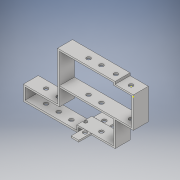
# Autodesk Inventor part: SENGH IS KENGH
Saved by Autodesk Inventor 2017 (Build 210142000, 142)
## iProperties
Created: 2017-11-30
Part Number: SENGH IS KENGH
Material: Generic
Document SubType Name: Modeling
Designer: Sam
Density: 1 g/cm^3
Appearance: Default
Author: Sam
Autodesk Inventor part; units mm, degrees
ref_plane "YZ Plane" through (0, 0, 0) normal (1, 0, 0) x (0, 1, 0)
ref_plane "XZ Plane" through (0, 0, 0) normal (0, 1, 0) x (-1, 0, 0)
ref_plane "XY Plane" through (0, 0, 0) normal (0, 0, 1) x (1, 0, 0)
sketch "Sketch1" plane through (0, 0, 0) normal (0, 0, 1) x (1, 0, 0)
  line L0 (0, 2) -> (0, 0) projected
  line L1 (0, 2) -> (-89, 2) projected
  line L2 (-89, 0) -> (-89, 2) projected
  line L3 (0, 0) -> (-89, 0) projected
  circle A0 centre (-28, -35.5) radius 1.5 projected
  circle A1 centre (-36, -35.5) radius 1.5 projected
  line L4 (-66, -36) -> (-40, -36) projected
  line L5 (-40, -36) -> (-40, -41) projected
  line L6 (-20.7846, -41) -> (-40, -41) projected
  line L7 (-20.7846, 0) -> (-20.7846, -41) projected
  line L8 (-20.7846, 0) -> (-22, 0) projected
  line L9 (-22, 0) -> (-22, -30) projected
  line L10 (-66, -31.5748) -> (-66, -36) projected
  line L11 (0, -41) -> (-20.7846, -41) projected
  line L12 (0, 0) -> (0, -41) projected
  line L13 (0, 0) -> (-20.7846, 0) projected
  line L14 (-20.7846, 0) -> (-20.7846, -41) projected
  line L15 (0, 46) -> (0, 0) projected
  circle A2 centre (-28, 45.5) radius 1.5 projected
  circle A3 centre (-36, 45.5) radius 1.5 projected
  circle A4 centre (-98, 52) radius 1.5 projected
  line L16 (-49.0437, 51) -> (-20.7846, 51) projected
  line L17 (-104, 55.8081) -> (-49.0437, 51) projected
  line L18 (-104, 55.8081) -> (-104, 48) projected
  line L19 (-104, 48) -> (-81, 48) projected
  line L20 (-81, 48) -> (-81, 42.8871) projected
  line L21 (-81, 42.8871) -> (-48, 40) projected
  line L22 (-48, 40) -> (-22, 40) projected
  line L23 (-22, 40) -> (-22, 46) projected
  line L24 (-22, 46) -> (-20.7846, 46) projected
  line L25 (-20.7846, 51) -> (-20.7846, 46) projected
  line L26 (-22, 46) -> (0, 46) projected
  line L27 (-22, 40) -> (-22, 46) projected
  line L28 (0, 40) -> (-22, 40) projected
  line L29 (0, 46) -> (0, 40) projected
  line L30 (-22, 0) -> (-22, -30)
  line L31 (-91.246, 40) -> (-22, 40)
  line L32 (-22, 40) -> (-22, 36.9892)
  line L33 (-22, 36.9892) -> (0, 36.9892)
  line L34 (0, 36.9892) -> (0, 2)
  line L35 (-23.9878, 0) -> (-24, 0)
  line L36 (-24, 0) -> (-23.8812, -27.9971)
  line L37 (-91, -18) -> (-114, -18) projected
  line L38 (-132.3701, 81.1945) -> (-132.3701, -67.1672)
  line L39 (-91, -18) -> (-132.3701, -18)
  line L40 (-132.3701, -18) -> (-132.3701, -29.4267)
  line L41 (-91, -18) -> (-91.246, 40)
  line L42 (-23.8812, -27.9971) -> (-68.0077, -28.1843)
  line L43 (-130.363, -20.001) -> (-88.993, -20.001)
  line L44 (-88.993, 37.9938) -> (-23.9878, 37.9938)
  line L45 (-23.9878, 37.9938) -> (-23.9878, 35.1472)
  line L46 (-23.9878, 35.1472) -> (-2.1372, 35.1472)
  line L47 (-2.1372, 35.1472) -> (-2.1372, 2)
  line L48 (-130.363, -20.001) -> (-130.363, -33.7874)
  line L49 (-130.363, -36) -> (-66, -36)
  line L50 (-132.3701, -18) -> (-132.3701, -36)
  line L51 (-132.3701, -36) -> (-130.363, -36)
  line L52 (-130.363, -33.7874) -> (-68, -33.7874)
  line L53 (-66, -33.7874) -> (-66, -36)
  line L54 (-66, -33.7874) -> (-66, -31.5748)
  line L55 (-68, -33.7874) -> (-68, -31.5748)
  line L56 (-68, -31.5748) -> (-68, -30)
  line L57 (-68, -30) -> (-68.0077, -28.1843)
  line L58 (-66, -30.1103) -> (-66, -31.5748)
  line L59 (-22, -30) -> (-66, -30)
  line L60 (-66, -30) -> (-66, -30.1103)
  line L61 (-2.1372, 2) -> (-89, 2)
  line L62 (0, 2) -> (0, 0)
  line L63 (0, 0) -> (-22, 0)
  line L64 (-24, 0) -> (-89, 0)
  line L65 (-88.993, -20.001) -> (-88.993, 0)
  line L66 (-88.993, 2) -> (-88.993, 37.9938)
  dimension "d0" = 2
  dimension "d1" = 27.9974
  dimension "d6" = 41.37
  dimension "d8" = 57.9948
  dimension "d10" = 65.0052
  dimension "d14" = 2
  constraints: 72 end point, 13 perpendicular, 11 point on line, 6 vertical, 4 collinear, 2 parallel, 1 horizontal, 1 midpoint, 2 other
  measures "d0" distance of L8.end L35.end
  measures "d1" distance of L35.end L36.end
  measures "d6" distance of L43.start L43.end
  measures "d8" distance of L43.end L44.start
  measures "d10" distance of L44.start L44.end
  measures "d14" distance of L52.end L53.start
extrude "Extrusion2" add sketch "Sketch1" against normal blind 18 contours L1 L47 L46 L45 L44 L66 L2 L3 L65 L43 L48 L52 L55 L56 L57 L42 L36 L9 L59 L60 L58 L10 L49 L51 L38 L39 L37 L41 L31 L22 L32 L33 L15
sketch "Sketch5" plane through (-23.9878, 35.1472, 0) normal (0, -1, 0) x (1, 0, 0)
  point P0 (23.9878, 0)
sketch "Sketch6" plane through (0, 0, -18) normal (0, 0, -1) x (-1, 0, 0)
  line L0 (22, -30) -> (66, -30) projected
  line L1 (68.0077, -28.1843) -> (23.8812, -27.9971) projected
  line L2 (66, -30) -> (46.9738, -30)
  line L3 (46.9738, -30) -> (46.9738, -28.0951)
  line L4 (46.9738, -28.0951) -> (66, -28.0951)
  line L5 (66, -28.0951) -> (66, -30)
  point P0 (0, 0)
  constraints: 8 end point, 2 parallel, 1 horizontal, 1 perpendicular, 1 point on line
extrude "Extrusion6" add sketch "Sketch6" along normal blind 25
sketch "Sketch7" plane through (-132.3701, -36, 0) normal (0, -1, 0) x (1, 0, 0)
  arc A0 (20.1763, -7.9629) -> (20.3806, -9.5438) centre (18.3701, -9) ccw
  spline S0 degree 3 number of poles 884
  arc A1 (63.5787, -11.8624) -> (67.8965, -12.5067) centre (66.2955, -8.4452) ccw
  arc A2 (67.8965, -12.5067) -> (70.6134, -9.0895) centre (66.2955, -8.4452) ccw
  arc A3 (70.6134, -9.0895) -> (69.0124, -5.028) centre (66.2955, -8.4452) ccw
  arc A4 (69.0124, -5.028) -> (64.6946, -4.3837) centre (66.2955, -8.4452) ccw
  arc A5 (64.6946, -4.3837) -> (61.9777, -7.8009) centre (66.2955, -8.4452) ccw
  arc A6 (61.9777, -7.8009) -> (63.5787, -11.8624) centre (66.2955, -8.4452) ccw
  arc A7 (67.9695, -7.2059) -> (66.6029, -6.3852) centre (66.2955, -8.4452) ccw
  arc A8 (66.6029, -6.3852) -> (67.9695, -7.2059) centre (66.2955, -8.4452) ccw
  arc A9 (73.8571, -24.1243) -> (78.1749, -24.7686) centre (76.574, -20.7071) ccw
  arc A10 (78.1749, -24.7686) -> (80.8918, -21.3514) centre (76.574, -20.7071) ccw
  arc A11 (80.8918, -21.3514) -> (79.2908, -17.2899) centre (76.574, -20.7071) ccw
  arc A12 (79.2908, -17.2899) -> (74.973, -16.6456) centre (76.574, -20.7071) ccw
  arc A13 (74.973, -16.6456) -> (72.2561, -20.0628) centre (76.574, -20.7071) ccw
  arc A14 (72.2561, -20.0628) -> (73.8571, -24.1243) centre (76.574, -20.7071) ccw
  arc A15 (78.2479, -19.4678) -> (76.8813, -18.6471) centre (76.574, -20.7071) ccw
  arc A16 (76.8813, -18.6471) -> (78.2479, -19.4678) centre (76.574, -20.7071) ccw
  spline S1 degree 3 number of poles 1000
  arc A17 (69.1532, -39.4172) -> (73.471, -40.0615) centre (71.8701, -36) ccw
  arc A18 (73.471, -40.0615) -> (76.1879, -36.6443) centre (71.8701, -36) ccw
  arc A19 (76.1879, -36.6443) -> (74.5869, -32.5828) centre (71.8701, -36) ccw
  arc A20 (74.5869, -32.5828) -> (70.2691, -31.9385) centre (71.8701, -36) ccw
  arc A21 (70.2691, -31.9385) -> (67.5522, -35.3557) centre (71.8701, -36) ccw
  arc A22 (67.5522, -35.3557) -> (69.1532, -39.4172) centre (71.8701, -36) ccw
  arc A23 (73.544, -34.7607) -> (72.1774, -33.94) centre (71.8701, -36) ccw
  arc A24 (72.1774, -33.94) -> (73.544, -34.7607) centre (71.8701, -36) ccw
  point P0 (132.3701, 0)
sketch "Sketch8" plane through (0, 0, 0) normal (0, 0, 1) x (1, 0, 0)
  line L0 (0, 2) -> (0, 36.9892) projected
  line L1 (0, 2) -> (-88.993, 2)
  line L2 (-88.993, 2) -> (-88.993, 0)
  line L3 (-88.993, 0) -> (0, 0)
  line L4 (0, 0) -> (0, 2)
  point P0 (0, 0)
  constraints: 8 end point, 2 parallel, 1 horizontal, 1 perpendicular
extrude "Extrusion7" add sketch "Sketch8" against normal blind 18
sketch "Sketch9" plane through (-23.9878, 35.1472, 0) normal (0, -1, 0) x (1, 0, 0)
  circle A0 centre (12.9653, -8.5) radius 1 projected
  point P0 (23.9878, 0)
sketch "Sketch10" plane through (-22, 36.9892, 0) normal (0, 1, 0) x (1, 0, 0)
  circle A0 centre (10.6789, 8.5163) radius 2.5
  point P0 (22, 0)
  dimension "d27" = 5
  constraints: 1 centre point
  measures "d27" diameter of A0
sketch "Sketch11" plane through (-23.9878, 35.1472, 0) normal (0, -1, 0) x (1, 0, 0)
  point P0 (23.9878, 0)
extrude "Extrusion8" cut sketch "Sketch10" against normal through all
sketch "Sketch12" plane through (-132.3701, -36, 0) normal (0, -1, 0) x (1, 0, 0)
  circle A0 centre (18.3329, -9.0632) radius 2.5
  circle A1 centre (66.3878, -8.536) radius 2.5
  point P0 (132.3701, 0)
  dimension "d30" = 5
  dimension "d31" = 5
  constraints: 2 centre point
  measures "d30" diameter of A0
  measures "d31" diameter of A1
extrude "Extrusion9" cut sketch "Sketch12" against normal through all contours A0
extrude "Extrusion10" cut sketch "Sketch7" against normal blind 25 contours A8 A7
sketch "Sketch14" plane through (-132.3701, -36, 0) normal (0, -1, 0) x (1, 0, 0)
  arc A0 (47.613, -10.8143) -> (51.9308, -11.4586) centre (50.3299, -7.3971) ccw projected
  arc A1 (51.9308, -11.4586) -> (54.6477, -8.0414) centre (50.3299, -7.3971) ccw projected
  arc A2 (54.6477, -8.0414) -> (53.0468, -3.9799) centre (50.3299, -7.3971) ccw projected
  arc A3 (53.0468, -3.9799) -> (48.7289, -3.3356) centre (50.3299, -7.3971) ccw projected
  arc A4 (48.7289, -3.3356) -> (46.0121, -6.7528) centre (50.3299, -7.3971) ccw projected
  arc A5 (46.0121, -6.7528) -> (47.613, -10.8143) centre (50.3299, -7.3971) ccw projected
  arc A6 (52.0039, -6.1578) -> (50.6373, -5.3371) centre (50.3299, -7.3971) ccw projected
  arc A7 (50.6373, -5.3371) -> (52.0039, -6.1578) centre (50.3299, -7.3971) ccw projected
  circle A8 centre (50.3299, -7.3971) radius 2.5
  point P0 (132.3701, 0)
  dimension "d39" = 5
  constraints: 1 centre point, 1 coincident
  measures "d39" diameter of A8
extrude "Extrusion12" cut sketch "Sketch14" against normal blind 5 contours A7 A6 | A8
sketch "Sketch15" plane through (-66, -30, 0) normal (0, -1, 0) x (1, 0, 0)
  circle A0 centre (19.9882, -7.5812) radius 1.4875 projected
  arc A1 (7.487, -24.1243) -> (11.8049, -24.7686) centre (10.2039, -20.7071) ccw projected
  arc A2 (11.8049, -24.7686) -> (14.5217, -21.3514) centre (10.2039, -20.7071) ccw projected
  arc A3 (14.5217, -21.3514) -> (12.9208, -17.2899) centre (10.2039, -20.7071) ccw projected
  arc A4 (12.9208, -17.2899) -> (8.6029, -16.6456) centre (10.2039, -20.7071) ccw projected
  arc A5 (8.6029, -16.6456) -> (5.8861, -20.0628) centre (10.2039, -20.7071) ccw projected
  arc A6 (5.8861, -20.0628) -> (7.487, -24.1243) centre (10.2039, -20.7071) ccw projected
  arc A7 (11.8779, -19.4678) -> (10.5113, -18.6471) centre (10.2039, -20.7071) ccw projected
  arc A8 (10.5113, -18.6471) -> (11.8779, -19.4678) centre (10.2039, -20.7071) ccw projected
  arc A9 (2.7831, -39.4172) -> (7.101, -40.0615) centre (5.5, -36) ccw projected
  arc A10 (7.101, -40.0615) -> (9.8178, -36.6443) centre (5.5, -36) ccw projected
  arc A11 (9.8178, -36.6443) -> (8.2169, -32.5828) centre (5.5, -36) ccw projected
  arc A12 (8.2169, -32.5828) -> (3.899, -31.9385) centre (5.5, -36) ccw projected
  arc A13 (3.899, -31.9385) -> (1.1822, -35.3557) centre (5.5, -36) ccw projected
  arc A14 (1.1822, -35.3557) -> (2.7831, -39.4172) centre (5.5, -36) ccw projected
  arc A15 (7.174, -34.7607) -> (5.8074, -33.94) centre (5.5, -36) ccw projected
  arc A16 (5.8074, -33.94) -> (7.174, -34.7607) centre (5.5, -36) ccw projected
  circle A17 centre (19.9882, -7.5812) radius 2.5
  circle A18 centre (10.2039, -20.7071) radius 2.5
  circle A19 centre (5.5, -36) radius 2.5
  point P0 (66, 0)
  dimension "d42" = 5
  dimension "d43" = 5
  dimension "d44" = 5
  constraints: 3 centre point, 3 coincident
  measures "d42" diameter of A17
  measures "d43" diameter of A18
  measures "d44" diameter of A19
extrude "Extrusion13" cut sketch "Sketch15" against normal blind 50 contours A0 | A8 A7 | A16 A15 | A17 | A18 | A19
sketch "Sketch17" plane through (-91.246, 40, 0) normal (0, 1, 0) x (1, 0, 0)
  circle A0 centre (62.2283, 8.0888) radius 2.5
  arc A1 (72.7505, 5.8875) -> (75.0997, 6.2647) centre (72.5002, 14.9506) ccw
  arc A2 (72.584, 5.204) -> (72.7505, 5.8875) centre (62.2283, 8.0888) ccw
  arc A3 (74.4965, 3.7887) -> (72.584, 5.204) centre (68.1934, -2.7285) ccw
  arc A4 (74.189, 2.9955) -> (74.4965, 3.7887) centre (62.2283, 8.0888) ccw
  arc A5 (71.8222, 3.2392) -> (74.189, 2.9955) centre (73.9261, 12.0582) ccw
  arc A6 (71.4845, 2.6221) -> (71.8222, 3.2392) centre (62.2283, 8.0888) ccw
  arc A7 (72.9655, 0.76) -> (71.4845, 2.6221) centre (65.1905, -3.9038) ccw
  arc A8 (72.4632, 0.0734) -> (72.9655, 0.76) centre (62.2283, 8.0888) ccw
  arc A9 (70.2402, 0.9213) -> (72.4632, 0.0734) centre (74.5549, 8.8954) ccw
  arc A10 (69.7542, 0.4127) -> (70.2402, 0.9213) centre (62.2283, 8.0888) ccw
  arc A11 (70.7028, -1.7693) -> (69.7542, 0.4127) centre (61.9856, -4.2618) ccw
  arc A12 (70.0399, -2.3025) -> (70.7028, -1.7693) centre (62.2283, 8.0888) ccw
  arc A13 (68.1121, -0.9081) -> (70.0399, -2.3025) centre (74.3436, 5.6775) ccw
  arc A14 (67.5111, -1.2736) -> (68.1121, -0.9081) centre (62.2283, 8.0888) ccw
  arc A15 (67.8626, -3.6268) -> (67.5111, -1.2736) centre (58.7973, -3.7782) ccw
  arc A16 (67.0843, -3.9702) -> (67.8626, -3.6268) centre (62.2283, 8.0888) ccw
  arc A17 (65.583, -2.1244) -> (67.0843, -3.9702) centre (73.3067, 2.624) ccw
  arc A18 (64.9079, -2.3219) -> (65.583, -2.1244) centre (62.2283, 8.0888) ccw
  arc A19 (64.6384, -4.6859) -> (64.9079, -2.3219) centre (55.8428, -2.4858) ccw
  arc A20 (63.7977, -4.8161) -> (64.6384, -4.6859) centre (62.2283, 8.0888) ccw
  arc A21 (62.8254, -2.6446) -> (63.7977, -4.8161) centre (71.5149, -0.0571) ccw
  arc A22 (62.1221, -2.6607) -> (62.8254, -2.6446) centre (62.2283, 8.0888) ccw
  arc A23 (61.25, -4.8744) -> (62.1221, -2.6607) centre (53.3235, -0.4728) ccw
  arc A24 (60.4042, -4.7826) -> (61.25, -4.8744) centre (62.2283, 8.0888) ccw
  arc A25 (60.027, -2.4334) -> (60.4042, -4.7826) centre (69.0901, -2.1831) ccw
  arc A26 (59.3435, -2.2669) -> (60.027, -2.4334) centre (62.2283, 8.0888) ccw
  arc A27 (57.9282, -4.1794) -> (59.3435, -2.2669) centre (51.411, 2.1236) ccw
  arc A28 (57.135, -3.8719) -> (57.9282, -4.1794) centre (62.2283, 8.0888) ccw
  arc A29 (57.3787, -1.5052) -> (57.135, -3.8719) centre (66.1977, -3.6091) ccw
  arc A30 (56.7616, -1.1675) -> (57.3787, -1.5052) centre (62.2283, 8.0888) ccw
  arc A31 (54.8995, -2.6485) -> (56.7616, -1.1675) centre (50.2357, 5.1266) ccw
  arc A32 (54.2129, -2.1461) -> (54.8995, -2.6485) centre (62.2283, 8.0888) ccw
  arc A33 (55.0608, 0.0769) -> (54.2129, -2.1461) centre (63.0349, -4.2378) ccw
  arc A34 (54.5522, 0.5628) -> (55.0608, 0.0769) centre (62.2283, 8.0888) ccw
  arc A35 (52.3702, -0.3858) -> (54.5522, 0.5628) centre (49.8777, 8.3314) ccw
  arc A36 (51.837, 0.2771) -> (52.3702, -0.3858) centre (62.2283, 8.0888) ccw
  arc A37 (53.2314, 2.205) -> (51.837, 0.2771) centre (59.817, -4.0266) ccw
  arc A38 (52.8659, 2.806) -> (53.2314, 2.205) centre (62.2283, 8.0888) ccw
  arc A39 (50.5127, 2.4545) -> (52.8659, 2.806) centre (50.3613, 11.5197) ccw
  arc A40 (50.1693, 3.2328) -> (50.5127, 2.4545) centre (62.2283, 8.0888) ccw
  arc A41 (52.0151, 4.734) -> (50.1693, 3.2328) centre (56.7635, -2.9897) ccw
  arc A42 (51.8176, 5.4092) -> (52.0151, 4.734) centre (62.2283, 8.0888) ccw
  arc A43 (49.4536, 5.6787) -> (51.8176, 5.4092) centre (51.6537, 14.4742) ccw
  arc A44 (49.3234, 6.5193) -> (49.4536, 5.6787) centre (62.2283, 8.0888) ccw
  arc A45 (51.4949, 7.4917) -> (49.3234, 6.5193) centre (54.0824, -1.1978) ccw
  arc A46 (51.4788, 8.195) -> (51.4949, 7.4917) centre (62.2283, 8.0888) ccw
  arc A47 (49.2651, 9.0671) -> (51.4788, 8.195) centre (53.6667, 16.9936) ccw
  arc A48 (49.3569, 9.9128) -> (49.2651, 9.0671) centre (62.2283, 8.0888) ccw
  arc A49 (51.7061, 10.29) -> (49.3569, 9.9128) centre (51.9564, 1.227) ccw
  arc A50 (51.8726, 10.9735) -> (51.7061, 10.29) centre (62.2283, 8.0888) ccw
  arc A51 (49.9601, 12.3889) -> (51.8726, 10.9735) centre (56.2631, 18.906) ccw
  arc A52 (50.2676, 13.182) -> (49.9601, 12.3889) centre (62.2283, 8.0888) ccw
  arc A53 (52.6343, 12.9384) -> (50.2676, 13.182) centre (50.5304, 4.1193) ccw
  arc A54 (52.972, 13.5555) -> (52.6343, 12.9384) centre (62.2283, 8.0888) ccw
  arc A55 (51.491, 15.4176) -> (52.972, 13.5555) centre (59.2661, 20.0813) ccw
  arc A56 (51.9934, 16.1042) -> (51.491, 15.4176) centre (62.2283, 8.0888) ccw
  arc A57 (54.2164, 15.2562) -> (51.9934, 16.1042) centre (49.9017, 7.2822) ccw
  arc A58 (54.7023, 15.7649) -> (54.2164, 15.2562) centre (62.2283, 8.0888) ccw
  arc A59 (53.7537, 17.9469) -> (54.7023, 15.7649) centre (62.4709, 20.4394) ccw
  arc A60 (54.4166, 18.48) -> (53.7537, 17.9469) centre (62.2283, 8.0888) ccw
  arc A61 (56.3445, 17.0856) -> (54.4166, 18.48) centre (50.1129, 10.5) ccw
  arc A62 (56.9455, 17.4512) -> (56.3445, 17.0856) centre (62.2283, 8.0888) ccw
  arc A63 (56.594, 19.8043) -> (56.9455, 17.4512) centre (65.6592, 19.9557) ccw
  arc A64 (57.3723, 20.1478) -> (56.594, 19.8043) centre (62.2283, 8.0888) ccw
  arc A65 (58.8735, 18.3019) -> (57.3723, 20.1478) centre (51.1498, 13.5536) ccw
  arc A66 (59.5487, 18.4995) -> (58.8735, 18.3019) centre (62.2283, 8.0888) ccw
  arc A67 (59.8182, 20.8634) -> (59.5487, 18.4995) centre (68.6137, 18.6634) ccw
  arc A68 (60.6588, 20.9937) -> (59.8182, 20.8634) centre (62.2283, 8.0888) ccw
  arc A69 (61.6312, 18.8222) -> (60.6588, 20.9937) centre (52.9417, 16.2347) ccw
  arc A70 (62.3345, 18.8383) -> (61.6312, 18.8222) centre (62.2283, 8.0888) ccw
  arc A71 (63.2066, 21.0519) -> (62.3345, 18.8383) centre (71.1331, 16.6504) ccw
  arc A72 (64.0523, 20.9602) -> (63.2066, 21.0519) centre (62.2283, 8.0888) ccw
  arc A73 (64.4295, 18.611) -> (64.0523, 20.9602) centre (55.3665, 18.3607) ccw
  arc A74 (65.113, 18.4445) -> (64.4295, 18.611) centre (62.2283, 8.0888) ccw
  arc A75 (66.5284, 20.357) -> (65.113, 18.4445) centre (73.0455, 14.0539) ccw
  arc A76 (67.3215, 20.0495) -> (66.5284, 20.357) centre (62.2283, 8.0888) ccw
  arc A77 (67.0779, 17.6827) -> (67.3215, 20.0495) centre (58.2588, 19.7866) ccw
  arc A78 (67.695, 17.345) -> (67.0779, 17.6827) centre (62.2283, 8.0888) ccw
  arc A79 (69.5571, 18.826) -> (67.695, 17.345) centre (74.2208, 11.051) ccw
  arc A80 (70.2437, 18.3237) -> (69.5571, 18.826) centre (62.2283, 8.0888) ccw
  arc A81 (69.3957, 16.1007) -> (70.2437, 18.3237) centre (61.4217, 20.4154) ccw
  arc A82 (69.9044, 15.6147) -> (69.3957, 16.1007) centre (62.2283, 8.0888) ccw
  arc A83 (72.0864, 16.5633) -> (69.9044, 15.6147) centre (74.5789, 7.8461) ccw
  arc A84 (72.6195, 15.9004) -> (72.0864, 16.5633) centre (62.2283, 8.0888) ccw
  arc A85 (71.2251, 13.9726) -> (72.6195, 15.9004) centre (64.6395, 20.2041) ccw
  arc A86 (71.5907, 13.3716) -> (71.2251, 13.9726) centre (62.2283, 8.0888) ccw
  arc A87 (73.9438, 13.7231) -> (71.5907, 13.3716) centre (74.0952, 4.6578) ccw
  arc A88 (74.2873, 12.9448) -> (73.9438, 13.7231) centre (62.2283, 8.0888) ccw
  arc A89 (72.4414, 11.4435) -> (74.2873, 12.9448) centre (67.6931, 19.1672) ccw
  arc A90 (72.639, 10.7684) -> (72.4414, 11.4435) centre (62.2283, 8.0888) ccw
  arc A91 (75.0029, 10.4989) -> (72.639, 10.7684) centre (72.8029, 1.7033) ccw
  arc A92 (75.1332, 9.6582) -> (75.0029, 10.4989) centre (62.2283, 8.0888) ccw
  arc A93 (72.9617, 8.6859) -> (75.1332, 9.6582) centre (70.3742, 17.3754) ccw
  arc A94 (72.9778, 7.9826) -> (72.9617, 8.6859) centre (62.2283, 8.0888) ccw
  arc A95 (75.1914, 7.1105) -> (72.9778, 7.9826) centre (70.7899, -0.816) ccw
  arc A96 (75.0997, 6.2647) -> (75.1914, 7.1105) centre (62.2283, 8.0888) ccw
  spline S0 degree 3 number of poles 974
  circle A97 centre (62.2283, 8.0888) radius 2.5
  point P0 (91.246, 0)
  point P1 (31.2814, 8.5962)
  dimension "d53" = 5
  constraints: 1 centre point, 1 coincident
  measures "d53" diameter of A97
extrude "Extrusion15" cut sketch "Sketch17" against normal blind 25 contours A0
sketch "Sketch18" plane through (-91.246, 40, 0) normal (0, 1, 0) x (1, 0, 0)
  arc A0 (38.5455, 4.5703) -> (40.7689, 5.3998) centre (37.5392, 10.6619) ccw projected
  arc A1 (40.7689, 5.3998) -> (41.2222, 4.9749) centre (44.2369, 8.6456) ccw projected
  arc A2 (41.2222, 4.9749) -> (40.5383, 2.7025) centre (46.6824, 2.0925) ccw projected
  arc A3 (40.5383, 2.7025) -> (41.3457, 2.2706) centre (44.2369, 8.6456) ccw projected
  arc A4 (41.3457, 2.2706) -> (42.8565, 4.1006) centre (37.4284, 7.043) ccw projected
  arc A5 (42.8565, 4.1006) -> (43.4615, 3.9593) centre (44.2369, 8.6456) ccw projected
  arc A6 (43.4615, 3.9593) -> (44.0054, 1.6494) centre (49.6313, 4.1932) ccw projected
  arc A7 (44.0054, 1.6494) -> (44.9206, 1.6791) centre (44.2369, 8.6456) ccw projected
  arc A8 (44.9206, 1.6791) -> (45.3139, 4.0193) centre (39.1419, 3.8534) ccw projected
  arc A9 (45.3139, 4.0193) -> (45.9085, 4.1995) centre (44.2369, 8.6456) ccw projected
  arc A10 (45.9085, 4.1995) -> (47.5345, 2.471) centre (51.1348, 7.4869) ccw projected
  arc A11 (47.5345, 2.471) -> (48.3122, 2.9543) centre (44.2369, 8.6456) ccw projected
  arc A12 (48.3122, 2.9543) -> (47.4827, 5.1776) centre (42.2206, 1.948) ccw projected
  arc A13 (47.4827, 5.1776) -> (47.9076, 5.631) centre (44.2369, 8.6456) ccw projected
  arc A14 (47.9076, 5.631) -> (50.18, 4.9471) centre (50.79, 11.0911) ccw projected
  arc A15 (50.18, 4.9471) -> (50.6119, 5.7544) centre (44.2369, 8.6456) ccw projected
  arc A16 (50.6119, 5.7544) -> (48.7819, 7.2652) centre (45.8395, 1.8371) ccw projected
  arc A17 (48.7819, 7.2652) -> (48.9232, 7.8702) centre (44.2369, 8.6456) ccw projected
  arc A18 (48.9232, 7.8702) -> (51.2331, 8.4141) centre (48.6893, 14.04) ccw projected
  arc A19 (51.2331, 8.4141) -> (51.2034, 9.3293) centre (44.2369, 8.6456) ccw projected
  arc A20 (51.2034, 9.3293) -> (48.8632, 9.7226) centre (49.0291, 3.5506) ccw projected
  arc A21 (48.8632, 9.7226) -> (48.683, 10.3172) centre (44.2369, 8.6456) ccw projected
  arc A22 (48.683, 10.3172) -> (50.4115, 11.9432) centre (45.3956, 15.5435) ccw projected
  arc A23 (50.4115, 11.9432) -> (49.9282, 12.721) centre (44.2369, 8.6456) ccw projected
  arc A24 (49.9282, 12.721) -> (47.7049, 11.8915) centre (50.9345, 6.6293) ccw projected
  arc A25 (47.7049, 11.8915) -> (47.2515, 12.3164) centre (44.2369, 8.6456) ccw projected
  arc A26 (47.2515, 12.3164) -> (47.9354, 14.5887) centre (41.7914, 15.1988) ccw projected
  arc A27 (47.9354, 14.5887) -> (47.1281, 15.0206) centre (44.2369, 8.6456) ccw projected
  arc A28 (47.1281, 15.0206) -> (45.6173, 13.1906) centre (51.0454, 10.2482) ccw projected
  arc A29 (45.6173, 13.1906) -> (45.0123, 13.3319) centre (44.2369, 8.6456) ccw projected
  arc A30 (45.0123, 13.3319) -> (44.4684, 15.6418) centre (38.8425, 13.0981) ccw projected
  arc A31 (44.4684, 15.6418) -> (43.5532, 15.6121) centre (44.2369, 8.6456) ccw projected
  arc A32 (43.5532, 15.6121) -> (43.1599, 13.2719) centre (49.3319, 13.4378) ccw projected
  arc A33 (43.1599, 13.2719) -> (42.5653, 13.0917) centre (44.2369, 8.6456) ccw projected
  arc A34 (42.5653, 13.0917) -> (40.9393, 14.8202) centre (37.339, 9.8043) ccw projected
  arc A35 (40.9393, 14.8202) -> (40.1615, 14.337) centre (44.2369, 8.6456) ccw projected
  arc A36 (40.1615, 14.337) -> (40.991, 12.1136) centre (46.2532, 15.3433) ccw projected
  arc A37 (40.991, 12.1136) -> (40.5661, 11.6603) centre (44.2369, 8.6456) ccw projected
  arc A38 (40.5661, 11.6603) -> (38.2938, 12.3442) centre (37.6837, 6.2001) ccw projected
  arc A39 (38.2938, 12.3442) -> (37.8619, 11.5368) centre (44.2369, 8.6456) ccw projected
  arc A40 (37.8619, 11.5368) -> (39.6919, 10.026) centre (42.6343, 15.4541) ccw projected
  arc A41 (39.6919, 10.026) -> (39.5506, 9.421) centre (44.2369, 8.6456) ccw projected
  arc A42 (39.5506, 9.421) -> (37.2407, 8.8771) centre (39.7844, 3.2512) ccw projected
  arc A43 (37.2407, 8.8771) -> (37.2704, 7.9619) centre (44.2369, 8.6456) ccw projected
  arc A44 (37.2704, 7.9619) -> (39.6106, 7.5686) centre (39.4447, 13.7406) ccw projected
  arc A45 (39.6106, 7.5686) -> (39.7908, 6.974) centre (44.2369, 8.6456) ccw projected
  arc A46 (39.7908, 6.974) -> (38.0623, 5.348) centre (43.0782, 1.7477) ccw projected
  arc A47 (38.0623, 5.348) -> (38.5455, 4.5703) centre (44.2369, 8.6456) ccw projected
  arc A48 (38.9325, 10.6393) -> (36.5568, 10.7286) centre (37.4538, 2.9388) ccw projected
  arc A49 (36.5568, 10.7286) -> (36.3051, 11.3561) centre (29.2448, 8.1601) ccw projected
  arc A50 (36.3051, 11.3561) -> (37.9607, 13.0623) centre (31.5707, 17.6067) ccw projected
  arc A51 (37.9607, 13.0623) -> (37.5003, 13.8032) centre (29.2448, 8.1601) ccw projected
  arc A52 (37.5003, 13.8032) -> (35.2373, 13.0745) centre (38.7445, 6.0613) ccw projected
  arc A53 (35.2373, 13.0745) -> (34.7862, 13.5781) centre (29.2448, 8.1601) ccw projected
  arc A54 (34.7862, 13.5781) -> (35.7585, 15.7477) centre (28.1995, 17.8326) ccw projected
  arc A55 (35.7585, 15.7477) -> (35.0724, 16.2865) centre (29.2448, 8.1601) ccw projected
  arc A56 (35.0724, 16.2865) -> (33.1951, 14.8277) centre (38.8894, 9.437) ccw projected
  arc A57 (33.1951, 14.8277) -> (32.5989, 15.1466) centre (29.2448, 8.1601) ccw projected
  arc A58 (32.5989, 15.1466) -> (32.7705, 17.5179) centre (24.9543, 16.8917) ccw projected
  arc A59 (32.7705, 17.5179) -> (31.9415, 17.7896) centre (29.2448, 8.1601) ccw projected
  arc A60 (31.9415, 17.7896) -> (30.6764, 15.7767) centre (37.871, 12.6587) ccw projected
  arc A61 (30.6764, 15.7767) -> (30.0071, 15.8725) centre (29.2448, 8.1601) ccw projected
  arc A62 (30.0071, 15.8725) -> (29.3573, 18.1594) centre (22.2267, 14.8977) ccw projected
  arc A63 (29.3573, 18.1594) -> (28.4854, 18.1312) centre (29.2448, 8.1601) ccw projected
  arc A64 (28.4854, 18.1312) -> (27.985, 15.807) centre (35.8122, 15.3377) ccw projected
  arc A65 (27.985, 15.807) -> (27.3233, 15.6681) centre (29.2448, 8.1601) ccw projected
  arc A66 (27.3233, 15.6681) -> (25.9306, 17.5949) centre (20.3455, 12.0911) ccw projected
  arc A67 (25.9306, 17.5949) -> (25.1209, 17.2701) centre (29.2448, 8.1601) ccw projected
  arc A68 (25.1209, 17.2701) -> (25.4456, 14.915) centre (32.9612, 17.151) ccw projected
  arc A69 (25.4456, 14.915) -> (24.8713, 14.5581) centre (29.2448, 8.1601) ccw projected
  arc A70 (24.8713, 14.5581) -> (22.9035, 15.8924) centre (19.5377, 8.8103) ccw projected
  arc A71 (22.9035, 15.8924) -> (22.2537, 15.3103) centre (29.2448, 8.1601) ccw projected
  arc A72 (22.2537, 15.3103) -> (23.3644, 13.2082) centre (29.662, 17.8799) ccw projected
  arc A73 (23.3644, 13.2082) -> (22.9468, 12.6765) centre (29.2448, 8.1601) ccw projected
  arc A74 (22.9468, 12.6765) -> (20.6413, 13.2572) centre (19.9007, 5.4511) ccw projected
  arc A75 (20.6413, 13.2572) -> (20.2298, 12.488) centre (29.2448, 8.1601) ccw projected
  arc A76 (20.2298, 12.488) -> (21.9924, 10.8925) centre (26.3124, 17.4364) ccw projected
  arc A77 (21.9924, 10.8925) -> (21.7819, 10.2501) centre (29.2448, 8.1601) ccw projected
  arc A78 (21.7819, 10.2501) -> (19.4168, 10.0073) centre (21.3908, 2.4186) ccw projected
  arc A79 (19.4168, 10.0073) -> (19.2932, 9.1437) centre (29.2448, 8.1601) ccw projected
  arc A80 (19.2932, 9.1437) -> (21.4952, 8.2473) centre (23.3166, 15.8741) ccw projected
  arc A81 (21.4952, 8.2473) -> (21.5171, 7.5716) centre (29.2448, 8.1601) ccw projected
  arc A82 (21.5171, 7.5716) -> (19.3778, 6.5346) centre (23.8281, 0.0786) ccw projected
  arc A83 (19.3778, 6.5346) -> (19.557, 5.6808) centre (29.2448, 8.1601) ccw projected
  arc A84 (19.557, 5.6808) -> (21.9328, 5.5916) centre (21.0357, 13.3813) ccw projected
  arc A85 (21.9328, 5.5916) -> (22.1844, 4.9641) centre (29.2448, 8.1601) ccw projected
  arc A86 (22.1844, 4.9641) -> (20.5288, 3.2579) centre (26.9188, -1.2866) ccw projected
  arc A87 (20.5288, 3.2579) -> (20.9892, 2.5169) centre (29.2448, 8.1601) ccw projected
  arc A88 (20.9892, 2.5169) -> (23.2522, 3.2456) centre (19.745, 10.2588) ccw projected
  arc A89 (23.2522, 3.2456) -> (23.7033, 2.742) centre (29.2448, 8.1601) ccw projected
  arc A90 (23.7033, 2.742) -> (22.731, 0.5725) centre (30.29, -1.5124) ccw projected
  arc A91 (22.731, 0.5725) -> (23.4171, 0.0336) centre (29.2448, 8.1601) ccw projected
  arc A92 (23.4171, 0.0336) -> (25.2944, 1.4924) centre (19.6001, 6.8831) ccw projected
  arc A93 (25.2944, 1.4924) -> (25.8906, 1.1735) centre (29.2448, 8.1601) ccw projected
  arc A94 (25.8906, 1.1735) -> (25.719, -1.1978) centre (33.5352, -0.5716) ccw projected
  arc A95 (25.719, -1.1978) -> (26.548, -1.4694) centre (29.2448, 8.1601) ccw projected
  arc A96 (26.548, -1.4694) -> (27.8131, 0.5434) centre (20.6185, 3.6615) ccw projected
  arc A97 (27.8131, 0.5434) -> (28.4824, 0.4476) centre (29.2448, 8.1601) ccw projected
  arc A98 (28.4824, 0.4476) -> (29.1322, -1.8393) centre (36.2628, 1.4224) ccw projected
  arc A99 (29.1322, -1.8393) -> (30.0041, -1.8111) centre (29.2448, 8.1601) ccw projected
  arc A100 (30.0041, -1.8111) -> (30.5045, 0.5131) centre (22.6773, 0.9824) ccw projected
  arc A101 (30.5045, 0.5131) -> (31.1662, 0.652) centre (29.2448, 8.1601) ccw projected
  arc A102 (31.1662, 0.652) -> (32.559, -1.2748) centre (38.144, 4.229) ccw projected
  arc A103 (32.559, -1.2748) -> (33.3686, -0.95) centre (29.2448, 8.1601) ccw projected
  arc A104 (33.3686, -0.95) -> (33.044, 1.4052) centre (25.5283, -0.8309) ccw projected
  arc A105 (33.044, 1.4052) -> (33.6182, 1.762) centre (29.2448, 8.1601) ccw projected
  arc A106 (33.6182, 1.762) -> (35.586, 0.4277) centre (38.9518, 7.5098) ccw projected
  arc A107 (35.586, 0.4277) -> (36.2358, 1.0098) centre (29.2448, 8.1601) ccw projected
  arc A108 (36.2358, 1.0098) -> (35.1251, 3.1119) centre (28.8275, -1.5598) ccw projected
  arc A109 (35.1251, 3.1119) -> (35.5427, 3.6437) centre (29.2448, 8.1601) ccw projected
  arc A110 (35.5427, 3.6437) -> (37.8482, 3.0629) centre (38.5888, 10.8691) ccw projected
  arc A111 (37.8482, 3.0629) -> (38.2597, 3.8321) centre (29.2448, 8.1601) ccw projected
  arc A112 (38.2597, 3.8321) -> (36.4971, 5.4276) centre (32.1771, -1.1163) ccw projected
  arc A113 (36.4971, 5.4276) -> (36.7076, 6.0701) centre (29.2448, 8.1601) ccw projected
  arc A114 (36.7076, 6.0701) -> (39.0727, 6.3128) centre (37.0987, 13.9015) ccw projected
  arc A115 (39.0727, 6.3128) -> (39.1963, 7.1764) centre (29.2448, 8.1601) ccw projected
  arc A116 (39.1963, 7.1764) -> (36.9943, 8.0728) centre (35.173, 0.446) ccw projected
  arc A117 (36.9943, 8.0728) -> (36.9724, 8.7486) centre (29.2448, 8.1601) ccw projected
  arc A118 (36.9724, 8.7486) -> (39.1118, 9.7856) centre (34.6614, 16.2415) ccw projected
  arc A119 (39.1118, 9.7856) -> (38.9325, 10.6393) centre (29.2448, 8.1601) ccw projected
  circle A120 centre (44.2369, 8.6456) radius 2.5
  circle A121 centre (44.2369, 8.6456) radius 2.5 projected
  circle A122 centre (29.2448, 8.1601) radius 2.5 projected
  point P0 (91.246, 0)
  dimension "d56" = 5
  constraints: 1 centre point, 1 coincident
  measures "d56" diameter of A120
extrude "Extrusion17" cut sketch "Sketch18" against normal blind 25 contours A120
sketch "Sketch19" plane through (-91.246, 40, 0) normal (0, 1, 0) x (1, 0, 0)
  arc A0 (38.9325, 10.6393) -> (36.5568, 10.7286) centre (37.4538, 2.9388) ccw projected
  arc A1 (36.5568, 10.7286) -> (36.3051, 11.3561) centre (29.2448, 8.1601) ccw projected
  arc A2 (36.3051, 11.3561) -> (37.9607, 13.0623) centre (31.5707, 17.6067) ccw projected
  arc A3 (37.9607, 13.0623) -> (37.5003, 13.8032) centre (29.2448, 8.1601) ccw projected
  arc A4 (37.5003, 13.8032) -> (35.2373, 13.0745) centre (38.7445, 6.0613) ccw projected
  arc A5 (35.2373, 13.0745) -> (34.7862, 13.5781) centre (29.2448, 8.1601) ccw projected
  arc A6 (34.7862, 13.5781) -> (35.7585, 15.7477) centre (28.1995, 17.8326) ccw projected
  arc A7 (35.7585, 15.7477) -> (35.0724, 16.2865) centre (29.2448, 8.1601) ccw projected
  arc A8 (35.0724, 16.2865) -> (33.1951, 14.8277) centre (38.8894, 9.437) ccw projected
  arc A9 (33.1951, 14.8277) -> (32.5989, 15.1466) centre (29.2448, 8.1601) ccw projected
  arc A10 (32.5989, 15.1466) -> (32.7705, 17.5179) centre (24.9543, 16.8917) ccw projected
  arc A11 (32.7705, 17.5179) -> (31.9415, 17.7896) centre (29.2448, 8.1601) ccw projected
  arc A12 (31.9415, 17.7896) -> (30.6764, 15.7767) centre (37.871, 12.6587) ccw projected
  arc A13 (30.6764, 15.7767) -> (30.0071, 15.8725) centre (29.2448, 8.1601) ccw projected
  arc A14 (30.0071, 15.8725) -> (29.3573, 18.1594) centre (22.2267, 14.8977) ccw projected
  arc A15 (29.3573, 18.1594) -> (28.4854, 18.1312) centre (29.2448, 8.1601) ccw projected
  arc A16 (28.4854, 18.1312) -> (27.985, 15.807) centre (35.8122, 15.3377) ccw projected
  arc A17 (27.985, 15.807) -> (27.3233, 15.6681) centre (29.2448, 8.1601) ccw projected
  arc A18 (27.3233, 15.6681) -> (25.9306, 17.5949) centre (20.3455, 12.0911) ccw projected
  arc A19 (25.9306, 17.5949) -> (25.1209, 17.2701) centre (29.2448, 8.1601) ccw projected
  arc A20 (25.1209, 17.2701) -> (25.4456, 14.915) centre (32.9612, 17.151) ccw projected
  arc A21 (25.4456, 14.915) -> (24.8713, 14.5581) centre (29.2448, 8.1601) ccw projected
  arc A22 (24.8713, 14.5581) -> (22.9035, 15.8924) centre (19.5377, 8.8103) ccw projected
  arc A23 (22.9035, 15.8924) -> (22.2537, 15.3103) centre (29.2448, 8.1601) ccw projected
  arc A24 (22.2537, 15.3103) -> (23.3644, 13.2082) centre (29.662, 17.8799) ccw projected
  arc A25 (23.3644, 13.2082) -> (22.9468, 12.6765) centre (29.2448, 8.1601) ccw projected
  arc A26 (22.9468, 12.6765) -> (20.6413, 13.2572) centre (19.9007, 5.4511) ccw projected
  arc A27 (20.6413, 13.2572) -> (20.2298, 12.488) centre (29.2448, 8.1601) ccw projected
  arc A28 (20.2298, 12.488) -> (21.9924, 10.8925) centre (26.3124, 17.4364) ccw projected
  arc A29 (21.9924, 10.8925) -> (21.7819, 10.2501) centre (29.2448, 8.1601) ccw projected
  arc A30 (21.7819, 10.2501) -> (19.4168, 10.0073) centre (21.3908, 2.4186) ccw projected
  arc A31 (19.4168, 10.0073) -> (19.2932, 9.1437) centre (29.2448, 8.1601) ccw projected
  arc A32 (19.2932, 9.1437) -> (21.4952, 8.2473) centre (23.3166, 15.8741) ccw projected
  arc A33 (21.4952, 8.2473) -> (21.5171, 7.5716) centre (29.2448, 8.1601) ccw projected
  arc A34 (21.5171, 7.5716) -> (19.3778, 6.5346) centre (23.8281, 0.0786) ccw projected
  arc A35 (19.3778, 6.5346) -> (19.557, 5.6808) centre (29.2448, 8.1601) ccw projected
  arc A36 (19.557, 5.6808) -> (21.9328, 5.5916) centre (21.0357, 13.3813) ccw projected
  arc A37 (21.9328, 5.5916) -> (22.1844, 4.9641) centre (29.2448, 8.1601) ccw projected
  arc A38 (22.1844, 4.9641) -> (20.5288, 3.2579) centre (26.9188, -1.2866) ccw projected
  arc A39 (20.5288, 3.2579) -> (20.9892, 2.5169) centre (29.2448, 8.1601) ccw projected
  arc A40 (20.9892, 2.5169) -> (23.2522, 3.2456) centre (19.745, 10.2588) ccw projected
  arc A41 (23.2522, 3.2456) -> (23.7033, 2.742) centre (29.2448, 8.1601) ccw projected
  arc A42 (23.7033, 2.742) -> (22.731, 0.5725) centre (30.29, -1.5124) ccw projected
  arc A43 (22.731, 0.5725) -> (23.4171, 0.0336) centre (29.2448, 8.1601) ccw projected
  arc A44 (23.4171, 0.0336) -> (25.2944, 1.4924) centre (19.6001, 6.8831) ccw projected
  arc A45 (25.2944, 1.4924) -> (25.8906, 1.1735) centre (29.2448, 8.1601) ccw projected
  arc A46 (25.8906, 1.1735) -> (25.719, -1.1978) centre (33.5352, -0.5716) ccw projected
  arc A47 (25.719, -1.1978) -> (26.548, -1.4694) centre (29.2448, 8.1601) ccw projected
  arc A48 (26.548, -1.4694) -> (27.8131, 0.5434) centre (20.6185, 3.6615) ccw projected
  arc A49 (27.8131, 0.5434) -> (28.4824, 0.4476) centre (29.2448, 8.1601) ccw projected
  arc A50 (28.4824, 0.4476) -> (29.1322, -1.8393) centre (36.2628, 1.4224) ccw projected
  arc A51 (29.1322, -1.8393) -> (30.0041, -1.8111) centre (29.2448, 8.1601) ccw projected
  arc A52 (30.0041, -1.8111) -> (30.5045, 0.5131) centre (22.6773, 0.9824) ccw projected
  arc A53 (30.5045, 0.5131) -> (31.1662, 0.652) centre (29.2448, 8.1601) ccw projected
  arc A54 (31.1662, 0.652) -> (32.559, -1.2748) centre (38.144, 4.229) ccw projected
  arc A55 (32.559, -1.2748) -> (33.3686, -0.95) centre (29.2448, 8.1601) ccw projected
  arc A56 (33.3686, -0.95) -> (33.044, 1.4052) centre (25.5283, -0.8309) ccw projected
  arc A57 (33.044, 1.4052) -> (33.6182, 1.762) centre (29.2448, 8.1601) ccw projected
  arc A58 (33.6182, 1.762) -> (35.586, 0.4277) centre (38.9518, 7.5098) ccw projected
  arc A59 (35.586, 0.4277) -> (36.2358, 1.0098) centre (29.2448, 8.1601) ccw projected
  arc A60 (36.2358, 1.0098) -> (35.1251, 3.1119) centre (28.8275, -1.5598) ccw projected
  arc A61 (35.1251, 3.1119) -> (35.5427, 3.6437) centre (29.2448, 8.1601) ccw projected
  arc A62 (35.5427, 3.6437) -> (37.8482, 3.0629) centre (38.5888, 10.8691) ccw projected
  arc A63 (37.8482, 3.0629) -> (38.2597, 3.8321) centre (29.2448, 8.1601) ccw projected
  arc A64 (38.2597, 3.8321) -> (36.4971, 5.4276) centre (32.1771, -1.1163) ccw projected
  arc A65 (36.4971, 5.4276) -> (36.7076, 6.0701) centre (29.2448, 8.1601) ccw projected
  arc A66 (36.7076, 6.0701) -> (39.0727, 6.3128) centre (37.0987, 13.9015) ccw projected
  arc A67 (39.0727, 6.3128) -> (39.1963, 7.1764) centre (29.2448, 8.1601) ccw projected
  arc A68 (39.1963, 7.1764) -> (36.9943, 8.0728) centre (35.173, 0.446) ccw projected
  arc A69 (36.9943, 8.0728) -> (36.9724, 8.7486) centre (29.2448, 8.1601) ccw projected
  arc A70 (36.9724, 8.7486) -> (39.1118, 9.7856) centre (34.6614, 16.2415) ccw projected
  arc A71 (39.1118, 9.7856) -> (38.9325, 10.6393) centre (29.2448, 8.1601) ccw projected
  circle A72 centre (29.2448, 8.1601) radius 2.5
  circle A73 centre (29.2448, 8.1601) radius 2.5 projected
  point P0 (91.246, 0)
  dimension "d62" = 5
  constraints: 1 centre point, 1 coincident
  measures "d62" diameter of A72
extrude "Extrusion18" cut sketch "Sketch19" against normal blind 55 contours A72
sketch "Sketch21" plane through (0, 0, 0) normal (0, 0, 1) x (1, 0, 0)
  line L0 (-59.9332, -30.1099) -> (-50.7566, -30.1099)
  line L1 (-50.7566, -30.1099) -> (-50.7566, -28.1112)
  line L2 (-50.7566, -28.1112) -> (-59.9332, -28.1112)
  line L3 (-59.9332, -28.1112) -> (-59.9332, -30.1099)
  point P0 (0, 0)
  constraints: 8 end point, 2 parallel, 1 horizontal, 1 perpendicular
extrude "Extrusion19" add sketch "Sketch21" along normal blind 15
sketch "Sketch22" plane through (-59.9332, -30.1099, 0) normal (0, -1, 0) x (1, 0, 0)
  arc A0 (7.2587, -3.1973) -> (8.8548, -4.958) centre (13.427, 0.7905) ccw projected
  arc A1 (8.8548, -4.958) -> (9.6284, -4.532) centre (4.9055, 3.1292) ccw projected
  arc A2 (9.6284, -4.532) -> (8.9939, -2.2418) centre (2.3259, -5.3225) ccw projected
  arc A3 (8.9939, -2.2418) -> (9.5006, -1.8152) centre (4.9055, 3.1292) ccw projected
  arc A4 (9.5006, -1.8152) -> (11.649, -2.8311) centre (13.6733, 4.2296) ccw projected
  arc A5 (11.649, -2.8311) -> (12.2007, -2.1414) centre (4.9055, 3.1292) ccw projected
  arc A6 (12.2007, -2.1414) -> (10.7381, -0.2685) centre (5.7566, -5.6663) ccw projected
  arc A7 (10.7381, -0.2685) -> (11.043, 0.3196) centre (4.9055, 3.1292) ccw projected
  arc A8 (11.043, 0.3196) -> (13.4166, 0.2032) centre (12.5848, 7.5011) ccw projected
  arc A9 (13.4166, 0.2032) -> (13.6624, 1.0515) centre (4.9055, 3.1292) ccw projected
  arc A10 (13.6624, 1.0515) -> (11.5943, 2.2222) centre (9.0577, -4.6711) ccw projected
  arc A11 (11.5943, 2.2222) -> (11.651, 2.8822) centre (4.9055, 3.1292) ccw projected
  arc A12 (11.651, 2.8822) -> (13.8885, 3.683) centre (10.3272, 10.1071) ccw projected
  arc A13 (13.8885, 3.683) -> (13.7909, 4.5608) centre (4.9055, 3.1292) ccw projected
  arc A14 (13.7909, 4.5608) -> (11.4323, 4.8509) centre (11.7267, -2.4883) ccw projected
  arc A15 (11.4323, 4.8509) -> (11.2321, 5.4824) centre (4.9055, 3.1292) ccw projected
  arc A16 (11.2321, 5.4824) -> (12.9928, 7.0785) centre (7.2442, 11.6507) ccw projected
  arc A17 (12.9928, 7.0785) -> (12.5667, 7.8521) centre (4.9055, 3.1292) ccw projected
  arc A18 (12.5667, 7.8521) -> (10.2766, 7.2175) centre (13.3572, 0.5496) ccw projected
  arc A19 (10.2766, 7.2175) -> (9.85, 7.7243) centre (4.9055, 3.1292) ccw projected
  arc A20 (9.85, 7.7243) -> (10.8658, 9.8727) centre (3.8051, 11.897) ccw projected
  arc A21 (10.8658, 9.8727) -> (10.1762, 10.4244) centre (4.9055, 3.1292) ccw projected
  arc A22 (10.1762, 10.4244) -> (8.3032, 8.9617) centre (13.701, 3.9803) ccw projected
  arc A23 (8.3032, 8.9617) -> (7.7151, 9.2667) centre (4.9055, 3.1292) ccw projected
  arc A24 (7.7151, 9.2667) -> (7.8315, 11.6403) centre (0.5336, 10.8085) ccw projected
  arc A25 (7.8315, 11.6403) -> (6.9832, 11.8861) centre (4.9055, 3.1292) ccw projected
  arc A26 (6.9832, 11.8861) -> (5.8125, 9.818) centre (12.7058, 7.2814) ccw projected
  arc A27 (5.8125, 9.818) -> (5.1526, 9.8747) centre (4.9055, 3.1292) ccw projected
  arc A28 (5.1526, 9.8747) -> (4.3517, 12.1121) centre (-2.0723, 8.5509) ccw projected
  arc A29 (4.3517, 12.1121) -> (3.4739, 12.0146) centre (4.9055, 3.1292) ccw projected
  arc A30 (3.4739, 12.0146) -> (3.1838, 9.6559) centre (10.5231, 9.9504) ccw projected
  arc A31 (3.1838, 9.6559) -> (2.5524, 9.4557) centre (4.9055, 3.1292) ccw projected
  arc A32 (2.5524, 9.4557) -> (0.9563, 11.2164) centre (-3.616, 5.4679) ccw projected
  arc A33 (0.9563, 11.2164) -> (0.1826, 10.7904) centre (4.9055, 3.1292) ccw projected
  arc A34 (0.1826, 10.7904) -> (0.8172, 8.5002) centre (7.4851, 11.5809) ccw projected
  arc A35 (0.8172, 8.5002) -> (0.3104, 8.0736) centre (4.9055, 3.1292) ccw projected
  arc A36 (0.3104, 8.0736) -> (-1.838, 9.0895) centre (-3.8623, 2.0288) ccw projected
  arc A37 (-1.838, 9.0895) -> (-2.3897, 8.3998) centre (4.9055, 3.1292) ccw projected
  arc A38 (-2.3897, 8.3998) -> (-0.927, 6.5269) centre (4.0544, 11.9247) ccw projected
  arc A39 (-0.927, 6.5269) -> (-1.232, 5.9388) centre (4.9055, 3.1292) ccw projected
  arc A40 (-1.232, 5.9388) -> (-3.6056, 6.0552) centre (-2.7738, -1.2427) ccw projected
  arc A41 (-3.6056, 6.0552) -> (-3.8514, 5.2069) centre (4.9055, 3.1292) ccw projected
  arc A42 (-3.8514, 5.2069) -> (-1.7833, 4.0362) centre (0.7533, 10.9295) ccw projected
  arc A43 (-1.7833, 4.0362) -> (-1.84, 3.3762) centre (4.9055, 3.1292) ccw projected
  arc A44 (-1.84, 3.3762) -> (-4.0774, 2.5754) centre (-0.5162, -3.8487) ccw projected
  arc A45 (-4.0774, 2.5754) -> (-3.9799, 1.6976) centre (4.9055, 3.1292) ccw projected
  arc A46 (-3.9799, 1.6976) -> (-1.6212, 1.4075) centre (-1.9156, 8.7467) ccw projected
  arc A47 (-1.6212, 1.4075) -> (-1.421, 0.776) centre (4.9055, 3.1292) ccw projected
  arc A48 (-1.421, 0.776) -> (-3.1817, -0.82) centre (2.5669, -5.3923) ccw projected
  arc A49 (-3.1817, -0.82) -> (-2.7557, -1.5937) centre (4.9055, 3.1292) ccw projected
  arc A50 (-2.7557, -1.5937) -> (-0.4655, -0.9591) centre (-3.5462, 5.7088) ccw projected
  arc A51 (-0.4655, -0.9591) -> (-0.0389, -1.4659) centre (4.9055, 3.1292) ccw projected
  arc A52 (-0.0389, -1.4659) -> (-1.0548, -3.6143) centre (6.0059, -5.6386) ccw projected
  arc A53 (-1.0548, -3.6143) -> (-0.3651, -4.166) centre (4.9055, 3.1292) ccw projected
  arc A54 (-0.3651, -4.166) -> (1.5079, -2.7033) centre (-3.89, 2.2781) ccw projected
  arc A55 (1.5079, -2.7033) -> (2.0959, -3.0083) centre (4.9055, 3.1292) ccw projected
  arc A56 (2.0959, -3.0083) -> (1.9795, -5.3819) centre (9.2774, -4.5501) ccw projected
  arc A57 (1.9795, -5.3819) -> (2.8278, -5.6277) centre (4.9055, 3.1292) ccw projected
  arc A58 (2.8278, -5.6277) -> (3.9985, -3.5596) centre (-2.8948, -1.023) ccw projected
  arc A59 (3.9985, -3.5596) -> (4.6585, -3.6163) centre (4.9055, 3.1292) ccw projected
  arc A60 (4.6585, -3.6163) -> (5.4593, -5.8537) centre (11.8834, -2.2925) ccw projected
  arc A61 (5.4593, -5.8537) -> (6.3371, -5.7562) centre (4.9055, 3.1292) ccw projected
  arc A62 (6.3371, -5.7562) -> (6.6272, -3.3975) centre (-0.712, -3.692) ccw projected
  arc A63 (6.6272, -3.3975) -> (7.2587, -3.1973) centre (4.9055, 3.1292) ccw projected
  circle A64 centre (4.9055, 3.1292) radius 2.5
  circle A65 centre (4.9055, 3.1292) radius 2.5 projected
  point P0 (59.9332, 0)
  dimension "d67" = 5
  constraints: 1 centre point, 1 coincident
  measures "d67" diameter of A64
extrude "Extrusion20" cut sketch "Sketch22" against normal blind 15 contours A64
sketch "Sketch23" plane through (-132.3701, -36, 0) normal (0, -1, 0) x (1, 0, 0)
  circle A0 centre (50.3299, -7.3971) radius 2.5 projected
  arc A1 (66.3701, -6.3637) -> (66.3701, -10.5267) centre (66.2955, -8.4452) ccw projected
  line L0 (66.3701, 0) -> (66.3701, -6.3637) projected
  line L1 (0, 0) -> (66.3701, 0) projected
  line L2 (0, 0) -> (0, -18) projected
  line L3 (66.3701, -18) -> (0, -18) projected
  line L4 (66.3701, -10.5267) -> (66.3701, -18) projected
  circle A2 centre (18.3329, -9.0632) radius 2.5 projected
  circle A3 centre (34.35, -8.1986) radius 2.5 projected
  arc A4 (25.7402, -10.8199) -> (28.1164, -10.7881) centre (26.8311, -3.5562) ccw projected
  arc A5 (28.1164, -10.7881) -> (28.4003, -11.3866) centre (34.35, -8.1986) ccw projected
  arc A6 (28.4003, -11.3866) -> (26.8719, -13.2063) centre (33.1865, -16.9582) ccw projected
  arc A7 (26.8719, -13.2063) -> (27.3987, -13.9152) centre (34.35, -8.1986) ccw projected
  arc A8 (27.3987, -13.9152) -> (29.5819, -12.9764) centre (25.6269, -6.787) ccw projected
  arc A9 (29.5819, -12.9764) -> (30.0732, -13.4208) centre (34.35, -8.1986) ccw projected
  arc A10 (30.0732, -13.4208) -> (29.3575, -15.6869) centre (36.6273, -16.7366) ccw projected
  arc A11 (29.3575, -15.6869) -> (30.1155, -16.1402) centre (34.35, -8.1986) ccw projected
  arc A12 (30.1155, -16.1402) -> (31.7733, -14.4374) centre (25.7507, -10.2326) ccw projected
  arc A13 (31.7733, -14.4374) -> (32.3972, -14.6599) centre (34.35, -8.1986) ccw projected
  arc A14 (32.3972, -14.6599) -> (32.6032, -17.0274) centre (39.7213, -15.2152) ccw projected
  arc A15 (32.6032, -17.0274) -> (33.477, -17.1561) centre (34.35, -8.1986) ccw projected
  arc A16 (33.477, -17.1561) -> (34.3569, -14.9486) centre (27.1837, -13.3686) ccw projected
  arc A17 (34.3569, -14.9486) -> (35.0185, -14.9154) centre (34.35, -8.1986) ccw projected
  arc A18 (35.0185, -14.9154) -> (36.1148, -17.0238) centre (41.9976, -12.6256) ccw projected
  arc A19 (36.1148, -17.0238) -> (36.9714, -16.8083) centre (34.35, -8.1986) ccw projected
  arc A20 (36.9714, -16.8083) -> (36.9395, -14.4321) centre (29.7076, -15.7175) ccw projected
  arc A21 (36.9395, -14.4321) -> (37.538, -14.1483) centre (34.35, -8.1986) ccw projected
  arc A22 (37.538, -14.1483) -> (39.3578, -15.6767) centre (43.1096, -9.362) ccw projected
  arc A23 (39.3578, -15.6767) -> (40.0666, -15.1498) centre (34.35, -8.1986) ccw projected
  arc A24 (40.0666, -15.1498) -> (39.1278, -12.9666) centre (32.9384, -16.9217) ccw projected
  arc A25 (39.1278, -12.9666) -> (39.5722, -12.4754) centre (34.35, -8.1986) ccw projected
  arc A26 (39.5722, -12.4754) -> (41.8383, -13.191) centre (42.8881, -5.9213) ccw projected
  arc A27 (41.8383, -13.191) -> (42.2916, -12.433) centre (34.35, -8.1986) ccw projected
  arc A28 (42.2916, -12.433) -> (40.5888, -10.7753) centre (36.384, -16.7978) ccw projected
  arc A29 (40.5888, -10.7753) -> (40.8113, -10.1514) centre (34.35, -8.1986) ccw projected
  arc A30 (40.8113, -10.1514) -> (43.1788, -9.9453) centre (41.3667, -2.8272) ccw projected
  arc A31 (43.1788, -9.9453) -> (43.3075, -9.0715) centre (34.35, -8.1986) ccw projected
  arc A32 (43.3075, -9.0715) -> (41.1, -8.1916) centre (39.52, -15.3649) ccw projected
  arc A33 (41.1, -8.1916) -> (41.0668, -7.5301) centre (34.35, -8.1986) ccw projected
  arc A34 (41.0668, -7.5301) -> (43.1752, -6.4337) centre (38.777, -0.5509) ccw projected
  arc A35 (43.1752, -6.4337) -> (42.9598, -5.5772) centre (34.35, -8.1986) ccw projected
  arc A36 (42.9598, -5.5772) -> (40.5835, -5.6091) centre (41.8689, -12.8409) ccw projected
  arc A37 (40.5835, -5.6091) -> (40.2997, -5.0105) centre (34.35, -8.1986) ccw projected
  arc A38 (40.2997, -5.0105) -> (41.8281, -3.1908) centre (35.5134, 0.5611) ccw projected
  arc A39 (41.8281, -3.1908) -> (41.3012, -2.4819) centre (34.35, -8.1986) ccw projected
  arc A40 (41.3012, -2.4819) -> (39.1181, -3.4207) centre (43.0731, -9.6101) ccw projected
  arc A41 (39.1181, -3.4207) -> (38.6268, -2.9764) centre (34.35, -8.1986) ccw projected
  arc A42 (38.6268, -2.9764) -> (39.3424, -0.7102) centre (32.0727, 0.3395) ccw projected
  arc A43 (39.3424, -0.7102) -> (38.5844, -0.2569) centre (34.35, -8.1986) ccw projected
  arc A44 (38.5844, -0.2569) -> (36.9267, -1.9597) centre (42.9493, -6.1645) ccw projected
  arc A45 (36.9267, -1.9597) -> (36.3028, -1.7372) centre (34.35, -8.1986) ccw projected
  arc A46 (36.3028, -1.7372) -> (36.0968, 0.6303) centre (28.9786, -1.1819) ccw projected
  arc A47 (36.0968, 0.6303) -> (35.223, 0.759) centre (34.35, -8.1986) ccw projected
  arc A48 (35.223, 0.759) -> (34.3431, -1.4486) centre (41.5163, -3.0285) ccw projected
  arc A49 (34.3431, -1.4486) -> (33.6815, -1.4817) centre (34.35, -8.1986) ccw projected
  arc A50 (33.6815, -1.4817) -> (32.5851, 0.6267) centre (26.7023, -3.7715) ccw projected
  arc A51 (32.5851, 0.6267) -> (31.7286, 0.4112) centre (34.35, -8.1986) ccw projected
  arc A52 (31.7286, 0.4112) -> (31.7605, -1.965) centre (38.9923, -0.6797) ccw projected
  arc A53 (31.7605, -1.965) -> (31.162, -2.2488) centre (34.35, -8.1986) ccw projected
  arc A54 (31.162, -2.2488) -> (29.3422, -0.7205) centre (25.5903, -7.0351) ccw projected
  arc A55 (29.3422, -0.7205) -> (28.6333, -1.2473) centre (34.35, -8.1986) ccw projected
  arc A56 (28.6333, -1.2473) -> (29.5721, -3.4305) centre (35.7616, 0.5246) ccw projected
  arc A57 (29.5721, -3.4305) -> (29.1278, -3.9217) centre (34.35, -8.1986) ccw projected
  arc A58 (29.1278, -3.9217) -> (26.8616, -3.2061) centre (25.8119, -10.4759) ccw projected
  arc A59 (26.8616, -3.2061) -> (26.4083, -3.9641) centre (34.35, -8.1986) ccw projected
  arc A60 (26.4083, -3.9641) -> (28.1111, -5.6218) centre (32.3159, 0.4007) ccw projected
  arc A61 (28.1111, -5.6218) -> (27.8886, -6.2457) centre (34.35, -8.1986) ccw projected
  arc A62 (27.8886, -6.2457) -> (25.5211, -6.4518) centre (27.3333, -13.5699) ccw projected
  arc A63 (25.5211, -6.4518) -> (25.3924, -7.3256) centre (34.35, -8.1986) ccw projected
  arc A64 (25.3924, -7.3256) -> (27.6, -8.2055) centre (29.18, -1.0322) ccw projected
  arc A65 (27.6, -8.2055) -> (27.6332, -8.867) centre (34.35, -8.1986) ccw projected
  arc A66 (27.6332, -8.867) -> (25.5247, -9.9634) centre (29.9229, -15.8462) ccw projected
  arc A67 (25.5247, -9.9634) -> (25.7402, -10.8199) centre (34.35, -8.1986) ccw projected
  circle A68 centre (34.35, -8.1986) radius 2.5
  point P0 (132.3701, 0)
  dimension "d70" = 5
  constraints: 1 centre point, 1 coincident
  measures "d70" diameter of A68
extrude "Extrusion21" cut sketch "Sketch23" against normal blind 25 contours A3
equation "\"d32\" = d31"
body "Solid2"
